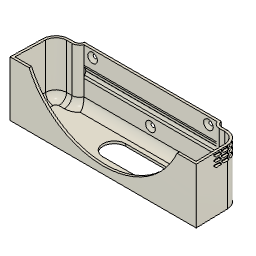
Helium Hotspot Vertical Stand (Autodesk Fusion 360 design; units mm, degrees)
Autodesk Fusion 360 part; units mm, degrees
sketch "Sketch1" plane through (0, 0, 0) normal (0, 1, 0) x (1, 0, 0)
  line L0 (75.5, 18.75) -> (-75.5, 18.75)
  line L1 (-75.5, 18.75) -> (-75.5, -18.75)
  line L2 (-75.5, -18.75) -> (75.5, -18.75)
  line L3 (75.5, -18.75) -> (75.5, 18.75)
  line L4 (75.5, 18.75) -> (-75.5, -18.75) construction
  line L5 (-75.5, 18.75) -> (75.5, -18.75) construction
  line L6 (0, 18.75) -> (0, -18.75)
  line L7 (75.5, 18.75) -> (55.5, 18.75)
  line L8 (55.5, 18.75) -> (55.5, 14.75)
  line L9 (55.5, 14.75) -> (75.5, 14.75)
  line L10 (75.5, 14.75) -> (75.5, 18.75)
  line L11 (-75.5, 18.75) -> (-55.5, 18.75)
  line L12 (-55.5, 18.75) -> (-55.5, 14.75)
  line L13 (-75.5, 14.75) -> (-75.5, 18.75)
  line L14 (-55.5, 14.75) -> (-75.5, 14.75)
  line L15 (-75.5, -18.75) -> (-74.5, 18.75)
  line L16 (75.5, -18.75) -> (74.5, 18.75)
  dimension "d1" = 151
  dimension "d2" = 37.5
  dimension "d3" = 20
  dimension "d4" = 4
  dimension "d11" = 1
  constraint horizontal L0
  constraint perpendicular L0 L1
  constraint parallel L0 L2
  constraint parallel L1 L3
  constraint coincident L4 origin
  constraint coincident L5 origin
  constraint midpoint L0 L6.start
  constraint midpoint L2 L6.end
  constraint horizontal L7
  constraint vertical L8
  constraint horizontal L9
  constraint vertical L10
  constraint symmetric L0.start L6 L0.end
  constraint symmetric L6 L7.end L11.end
  constraint symmetric L6 L8.end L12.end
  constraint symmetric L6 L9.end L13.start
  constraint coincident L11 L15.end
  constraint symmetric L1.end L6 L2.end
  constraint symmetric L6 L15.end L16.end
  measures "d1" distance of L1.end L2.end
  measures "d2" distance of L0.end L1.end
  measures "d3" distance of L0.start L7.end
  measures "d4" distance of L0.start L9.end
  measures "d11" distance of L0.end L15.end
extrude "Extrude1" add sketch "Sketch1" along normal blind 44 contours L0 L2 L6 L8 L9 L16 | L0 L2 L6 L12 L14 L15
fillet "Fillet1" radius 6.35 2 edges at (55.5, 22, -14.75) (-55.5, 22, -14.75)
fillet "Fillet2" radius 8.89 2 edges at (74.6067, 22, -14.75) (-74.6067, 22, -14.75)
shell "Shell1" thickness 2 outward yes removed faces 1 at (18.8166, 44, 6.7927)
sketch "Sketch2" plane through (0, 0, 20.75) normal (0, 0, 1) x (1, 0, 0)
  line L0 (-77.554, -2) -> (77.554, -2)
  line L1 (77.554, -2) -> (77.554, 44)
  line L2 (77.554, 44) -> (-77.554, 44)
  line L3 (-77.554, 44) -> (-77.554, -2)
  circle A0 centre (0, 71.5) radius 67.5
  dimension "d15" = 135
  dimension "d16" = 73.5
  measures "d15" diameter of A0
  measures "d16" distance of L0 A0.centre
extrude "Extrude2" cut sketch "Sketch2" against normal blind 25.4 contours L2 A0 picked at (14.1675, 25.9849)
sketch "Sketch3" plane through (0, 0, -18.75) normal (0, 0, 1) x (1, 0, 0)
  line L0 (-55.5, 0) -> (55.5, 0)
  line L1 (55.5, 0) -> (55.5, 44)
  line L2 (55.5, 44) -> (-55.5, 44)
  line L3 (-55.5, 44) -> (-55.5, 0)
  line L4 (-55.5, 28) -> (55.5, 28)
  line L5 (55.5, 28) -> (55.5, 21)
  line L6 (55.5, 21) -> (-55.5, 21)
  line L7 (-55.5, 21) -> (-55.5, 28)
  dimension "d19" = 7
  dimension "d20" = 21
  constraint horizontal L4
  constraint vertical L5
  constraint horizontal L6
  constraint vertical L7
  constraint coincident L3 L4.start
  measures "d19" distance of L4.start L6.end
  measures "d20" distance of L0 L6
extrude "Extrude3" cut sketch "Sketch3" against normal blind 1.5 contours L1 L3 L4 L5 L6 L7
fillet "Fillet3" radius 4.699 2 edges at (0, 21, -20.25) (0, 28, -20.25)
fillet "Fillet4" radius 3.302 2 edges at (0, 28, -18.75) (0, 21, -18.75)
sketch "Sketch4" plane through (0, 0, -18.75) normal (0, 0, 1) x (1, 0, 0)
  line L0 (-55.5, 29.2221) -> (55.5, 29.2221)
  line L1 (55.5, 29.2221) -> (55.5, 44)
  line L2 (55.5, 44) -> (-55.5, 44)
  line L3 (-55.5, 44) -> (-55.5, 29.2221)
  circle A0 centre (-48.26, 38.1) radius 1.5
  line L4 (0, 44) -> (0, -2.54)
  circle A1 centre (0, 12.7) radius 1.5
  circle A2 centre (48.26, 38.1) radius 1.5
  dimension "d27" = 3
  dimension "d28" = 3
  constraint midpoint L2 L4.start
  constraint perpendicular L2 L4
  constraint coincident L4 A1.centre
  constraint symmetric A0 L4 A2
  measures "d27" diameter of A0
  measures "d28" diameter of A1
extrude "Extrude4" cut sketch "Sketch4" against normal blind 2.54 contours A0 | L4 A1 | L4 A1 | A2
chamfer "Chamfer1" distance 2.5 distance2 2 3 edges at (-49.6585, 38.6424, -18.75) (-1.3985, 13.2424, -18.75) (46.8615, 38.6424, -18.75) measured on face at (15.7749, 31.7905, -18.75) measured on face at (-37.4944, 10.7515, -18.75) measured on face at (15.7749, 31.7905, -18.75)
fillet "Fillet5" radius 6.35 9 edges at (0, 0, -18.75) (57.8354, 0, -15.8443) (63.6749, 0, -14.75) (72.1524, 0, -12.2294) (75.1687, 0, 6.3265) (-75.1687, 0, 6.3265) (-72.1524, 0, -12.2294) (-63.6749, 0, -14.75) (-57.8354, 0, -15.8443)
sketch "Sketch5" plane through (76.946, 0, -2.0519) normal (0.999645, 0, -0.026657) x (-0.026657, 0, -0.999645)
  line L0 (4.0999, -2) -> (4.0999, 44)
  line L1 (4.0999, 44) -> (-22.81, 44)
  line L2 (-22.81, 44) -> (-22.81, -2)
  line L3 (-22.81, -2) -> (4.0999, -2)
  line L4 (-1.1969, 42.8953) -> (-7.5469, 42.8953)
  line L5 (-7.5469, 42.8953) -> (-7.5469, 40.3553)
  line L6 (-7.5469, 40.3553) -> (-1.1969, 40.3553)
  line L7 (-1.1969, 40.3553) -> (-1.1969, 42.8953)
  line L8 (-0.9429, 40.3553) -> (5.4071, 40.3553)
  line L9 (5.4071, 40.3553) -> (5.4071, 42.8953)
  line L10 (-0.9429, 42.8953) -> (-0.9429, 40.3553)
  line L11 (5.4071, 42.8953) -> (-0.9429, 42.8953)
  line L12 (5.6611, 40.3553) -> (12.0111, 40.3553)
  line L13 (12.0111, 40.3553) -> (12.0111, 42.8953)
  line L14 (5.6611, 42.8953) -> (5.6611, 40.3553)
  line L15 (12.0111, 42.8953) -> (5.6611, 42.8953)
  line L16 (-7.5469, 36.5453) -> (-1.1969, 36.5453)
  line L17 (-1.1969, 36.5453) -> (-1.1969, 39.0853)
  line L18 (-7.5469, 39.0853) -> (-7.5469, 36.5453)
  line L19 (-1.1969, 39.0853) -> (-7.5469, 39.0853)
  line L20 (-0.9429, 36.5453) -> (5.4071, 36.5453)
  line L21 (5.4071, 36.5453) -> (5.4071, 39.0853)
  line L22 (-0.9429, 39.0853) -> (-0.9429, 36.5453)
  line L23 (5.4071, 39.0853) -> (-0.9429, 39.0853)
  line L24 (5.6611, 36.5453) -> (12.0111, 36.5453)
  line L25 (12.0111, 36.5453) -> (12.0111, 39.0853)
  line L26 (5.6611, 39.0853) -> (5.6611, 36.5453)
  line L27 (12.0111, 39.0853) -> (5.6611, 39.0853)
  line L28 (-7.5469, 32.7353) -> (-1.1969, 32.7353)
  line L29 (-1.1969, 32.7353) -> (-1.1969, 35.2753)
  line L30 (-7.5469, 35.2753) -> (-7.5469, 32.7353)
  line L31 (-1.1969, 35.2753) -> (-7.5469, 35.2753)
  line L32 (-0.9429, 32.7353) -> (5.4071, 32.7353)
  line L33 (5.4071, 32.7353) -> (5.4071, 35.2753)
  line L34 (-0.9429, 35.2753) -> (-0.9429, 32.7353)
  line L35 (5.4071, 35.2753) -> (-0.9429, 35.2753)
  line L36 (5.6611, 32.7353) -> (12.0111, 32.7353)
  line L37 (12.0111, 32.7353) -> (12.0111, 35.2753)
  line L38 (5.6611, 35.2753) -> (5.6611, 32.7353)
  line L39 (12.0111, 35.2753) -> (5.6611, 35.2753)
  dimension "d48" = 6.604
  dimension "d49" = -3.81
  dimension "d50" = 2.54
  dimension "d51" = 6.35
  constraint horizontal L4
  constraint vertical L5
  constraint horizontal L6
  constraint vertical L7
  measures "d50" distance of L4.end L5.end
  measures "d51" distance of L5 L7
extrude "Extrude5" cut sketch "Sketch5" against normal blind 10.16 contours L0 L32 L34 L35 | L0 L32 L33 L35 | L0 L20 L22 L23 | L0 L20 L21 L23 | L0 L8 L9 L11 | L0 L8 L10 L11 | L4 L5 L6 L7 | L12 L13 L14 L15 | L16 L17 L18 L19 | L24 L25 L26 L27 | L28 L29 L30 L31 | L36 L37 L38 L39
chamfer "Chamfer2" distance 1.778 angle 45 18 edges at (76.1475, 32.7353, 5.519) (76.1475, 36.5453, 5.519) (76.1475, 40.3553, 5.519) (75.9715, 32.7353, -1.0826) (75.9715, 36.5453, -1.0826) (75.9715, 40.3553, -1.0826) (75.6702, 40.3553, -7.681) (75.6702, 36.5453, -7.681) (75.6702, 32.7353, -7.681) (75.9783, 42.8953, -0.8287) (75.7146, 42.8953, -7.4281) (71.5071, 42.8953, -13.9222) (71.5071, 39.0853, -13.9222) (71.5071, 35.2753, -13.9222) (75.7146, 35.2753, -7.4281) (75.7146, 39.0853, -7.4281) (75.9783, 39.0853, -0.8287) (75.9783, 35.2753, -0.8287)
fillet "Fillet6" [suppressed]
fillet "Fillet7" [suppressed]
sketch "Sketch6" plane through (0, -2, 0) normal (0, -1, 0) x (1, 0, 0)
  arc A0 (-76.8367, -6.1503) -> (-65.9506, -16.75) centre (-65.9506, -5.86) ccw
  line L0 (-65.9506, -16.75) -> (-61.3992, -16.75)
  arc A1 (-57.0633, -20.75) -> (-61.3992, -16.75) centre (-61.3992, -21.1) ccw
  line L1 (-57.0633, -20.75) -> (57.0633, -20.75)
  arc A2 (61.3992, -16.75) -> (57.0633, -20.75) centre (61.3992, -21.1) ccw
  line L2 (61.3992, -16.75) -> (65.9506, -16.75)
  arc A3 (65.9506, -16.75) -> (76.8367, -6.1503) centre (65.9506, -5.86) ccw
  line L3 (76.8367, -6.1503) -> (77.554, 20.75)
  line L4 (77.554, 20.75) -> (-77.554, 20.75)
  line L5 (-77.554, 20.75) -> (-76.8367, -6.1503)
  line L6 (-10.6852, -8.75) -> (41.5081, -8.75)
  arc A4 (41.5081, -8.75) -> (41.5081, 10.25) centre (41.5081, 0.75) ccw
  line L7 (41.5081, 10.25) -> (-10.6852, 10.25)
  arc A5 (-10.6852, 10.25) -> (-10.6852, -8.75) centre (-10.6852, 0.75) ccw
  line L8 (-10.6852, 0.75) -> (41.5081, 0.75) construction
  dimension "d52" = 19
  dimension "d53" = 35.5
  dimension "d54" = 21.5
  constraint tangent L6 A4
  constraint tangent A4 L7
  constraint parallel L6 L7
  constraint tangent L7 A5
  constraint tangent L6 A5
  constraint horizontal L8
  measures "d52" diameter of A4
  measures "d53" distance of L3 A4.centre
  measures "d54" distance of L1 A5.centre
extrude "Extrude6" cut sketch "Sketch6" against normal up to surface (2 mm away) contours L6 A4 L7 A5
fillet "Fillet8" [suppressed]
equation "d16 = 135 mm / 2 + 6 mm"
equation "d53 = 26 mm + ( 19 mm / 2 )"
equation "d54 = 12 mm + ( 19 mm / 2 )"
